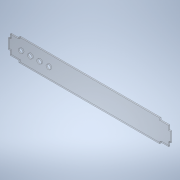
# Autodesk Inventor part: 103.013.01_Abdeckung_Gestell_hinten
Saved by Autodesk Inventor 2021 (Build 250183000, 183)
## iProperties
Created: 2021-11-25
Part Number: 103.013.01_Abdeckung_Gestell_hinten
Material: PMMA-Kunststoff
Document SubType Name: Modeling
Designer: Sebastian Seewald
Mass: 65.5279 g
Surface Area: 298.591 cm^2
Volume: 55.1582 cm^3
Density: 1.188 g/cm^3
Appearance: Polycarbonat - klar
Author: Sebastian Seewald
Autodesk Inventor part; units mm, degrees
ref_plane "YZ Plane" through (0, 0, 0) normal (1, 0, 0) x (0, 1, 0)
ref_plane "XZ Plane" through (0, 0, 0) normal (0, 1, 0) x (-1, 0, 0)
ref_plane "XY Plane" through (0, 0, 0) normal (0, 0, 1) x (1, 0, 0)
sketch "Skizze1" plane through (0, 0, 0) normal (0, 0, 1) x (1, 0, 0)
  line L0 (0, 0) -> (526.5, 0)
  line L1 (526.5, 0) -> (526.5, 72.5)
  line L2 (526.5, 72.5) -> (0, 72.5)
  line L3 (0, 72.5) -> (0, 0)
  line L4 (0, 72.5) -> (35, 72.5)
  line L5 (35, 72.5) -> (35, 66.15)
  line L6 (35, 66.15) -> (0, 66.15)
  line L7 (0, 66.15) -> (0, 72.5)
  line L8 (0, 72.5) -> (6.35, 72.5)
  line L9 (6.35, 72.5) -> (6.35, 52.5)
  line L10 (6.35, 52.5) -> (0, 52.5)
  line L11 (0, 52.5) -> (0, 72.5)
  line L12 (0, 36.25) -> (526.5, 36.25) construction
  line L13 (263.25, 72.5) -> (263.25, 0) construction
  line L14 (0, 0) -> (35, 0)
  line L15 (35, 0) -> (35, 6.35)
  line L16 (35, 6.35) -> (0, 6.35)
  line L17 (0, 6.35) -> (0, 0)
  line L18 (0, 0) -> (6.35, 0)
  line L19 (6.35, 0) -> (6.35, 20)
  line L20 (6.35, 20) -> (0, 20)
  line L21 (0, 20) -> (0, 0)
  line L22 (526.5, 72.5) -> (526.5, 0)
  line L23 (526.5, 72.5) -> (491.5, 72.5)
  line L24 (491.5, 72.5) -> (491.5, 66.15)
  line L25 (491.5, 66.15) -> (526.5, 66.15)
  line L26 (526.5, 66.15) -> (526.5, 72.5)
  line L27 (526.5, 72.5) -> (520.15, 72.5)
  line L28 (520.15, 72.5) -> (520.15, 52.5)
  line L29 (520.15, 52.5) -> (526.5, 52.5)
  line L30 (526.5, 52.5) -> (526.5, 72.5)
  line L31 (526.5, 0) -> (520.15, 0)
  line L32 (526.5, 0) -> (491.5, 0)
  line L33 (491.5, 0) -> (491.5, 6.35)
  line L34 (491.5, 6.35) -> (526.5, 6.35)
  line L35 (520.15, 0) -> (520.15, 20)
  line L36 (526.5, 6.35) -> (526.5, 0)
  line L37 (520.15, 20) -> (526.5, 20)
  line L38 (526.5, 20) -> (526.5, 0)
  point P0 (520.15, 66.15)
  point P1 (6.35, 66.15)
  point P2 (0, 52.5)
  point P3 (0, 20)
  point P4 (6.35, 6.35)
  point P5 (491.5, 0)
  point P6 (520.15, 6.35)
  point P7 (526.5, 20)
  dimension "d0" = 526.5
  dimension "d1" = 72.5
  dimension "d2" = 35
  dimension "d3" = 6.35
  dimension "d4" = 6.35
  dimension "d5" = 20
  constraints: 78 end point, 18 symmetric about line, 6 parallel, 4 midpoint, 3 horizontal, 3 perpendicular
  measures "d0" distance of L1.end L2.end
  measures "d1" distance between parallel lines of L0 L2
  measures "d2" distance between parallel lines of L3 L5
  measures "d3" distance between parallel lines of L2 L6
  measures "d4" distance between parallel lines of L3 L9
  measures "d5" distance between parallel lines of L2 L10
extrude "Extrusion1" add sketch "Skizze1" along normal blind 4 contours L15 L16 L19 L20 L3 L10 L9 L6 L5 L2 L24 L25 L28 L29 L1 L37 L35 L34 L33 L0
sketch "Skizze2" plane through (0, 0, 4) normal (0, 0, 1) x (1, 0, 0)
  circle A0 centre (40, 35) radius 7.5
  circle A1 centre (70, 35) radius 7.5
  circle A2 centre (100, 35) radius 7.5
  circle A3 centre (130, 35) radius 7.5
  line L0 (35, 0) -> (491.5, 0) projected
  line L1 (0, 52.5) -> (0, 20) projected
  point P0 (0, 0)
  dimension "d8" = 15
  dimension "d9" = 15
  dimension "d10" = 15
  dimension "d11" = 15
  dimension "d12" = 35
  dimension "d13" = 30
  dimension "d14" = 40
  dimension "d15" = 30
  dimension "d16" = 30
  constraints: 4 centre point, 3 horizontal alignment
  measures "d8" diameter of A3
  measures "d9" diameter of A2
  measures "d10" diameter of A1
  measures "d11" diameter of A0
  measures "d12" distance from line of L0 A0.centre
  measures "d13" distance of A0.centre A1.centre
  measures "d14" distance from line of L1 A0.centre
  measures "d15" distance of A1.centre A2.centre
  measures "d16" distance of A2.centre A3.centre
extrude "Extrusion2" cut sketch "Skizze2" against normal blind 10
